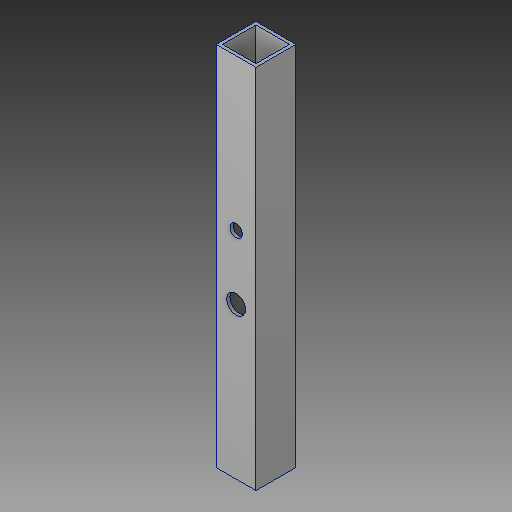
# Autodesk Inventor part: C010
Saved by Autodesk Inventor 2017 SP1 (Build 210196100, 196)
## iProperties
Created: 2017-06-14
Part Number: C010
Material: Aluminum 6061
Document SubType Name: Modeling
Designer: zallen
Density: 2.7 g/cm^3
Appearance: Aluminum - Flat
Description: 175 mm
Author: zallen
Autodesk Inventor part; units mm, degrees
ref_plane "YZ Plane" through (0, 0, 0) normal (1, 0, 0) x (0, 1, 0)
ref_plane "XZ Plane" through (0, 0, 0) normal (0, 1, 0) x (-1, 0, 0)
ref_plane "XY Plane" through (0, 0, 0) normal (0, 0, 1) x (1, 0, 0)
sketch "Sketch1" plane through (0, 0, 0) normal (0, 0, 1) x (1, 0, 0)
  line L0 (0, 0) -> (19, 0)
  line L1 (19, 0) -> (19, 175)
  line L2 (19, 175) -> (0, 175)
  line L3 (0, 175) -> (0, 0)
  dimension "d0" = 19
  dimension "d1" = 175
  constraints: 8 end point, 2 parallel, 1 horizontal, 1 perpendicular
  measures "d0" distance of L2.end L1.end
  measures "d1" distance of L1.end L0.end
extrude "Extrusion1" add sketch "Sketch1" along normal blind 19
sketch "Sketch2" plane through (0, 0, 0) normal (0, -1, 0) x (1, 0, 0)
  line L0 (0, 0) -> (19, 0) projected
  line L1 (19, 0) -> (19, 19) projected
  line L2 (0, 19) -> (19, 19) projected
  line L3 (0, 0) -> (0, 19) projected
  line L4 (17.5, 17.5) -> (17.5, 1.5)
  line L5 (17.5, 1.5) -> (1.5, 1.5)
  line L6 (1.5, 1.5) -> (1.5, 17.5)
  line L7 (1.5, 17.5) -> (17.5, 17.5)
  dimension "d4" = 1.5
  constraints: 8 end point, 3 other
  measures "d4" distance between parallel lines of L2 L7
extrude "Extrusion2" cut sketch "Sketch2" against normal through all contours L4 L5 L6 L7
sketch "Sketch3" plane through (0, 0, 19) normal (0, 0, 1) x (1, 0, 0)
  line L0 (9.5, 72.25) -> (9.5, 102.75) construction
  circle A0 centre (9.5, 102.75) radius 3
  circle A1 centre (9.5, 72.25) radius 4.5
  line L1 (19, 0) -> (19, 175) projected
  line L2 (19, 175) -> (0, 175) projected
  point P0 (0, 0)
  point P1 (19, 87.5)
  point P2 (9.5, 87.5)
  point P3 (9.5, 175)
  dimension "d7" = 30.5
  dimension "d8" = 6
  dimension "d9" = 9
  constraints: 3 midpoint, 2 centre point, 2 coincident, 2 end point, 1 horizontal alignment, 1 vertical, 1 vertical alignment
  measures "d7" distance of L0.start L0.end
  measures "d8" diameter of A0
  measures "d9" diameter of A1
extrude "Extrusion3" cut sketch "Sketch3" against normal through all
body "Solid1"
